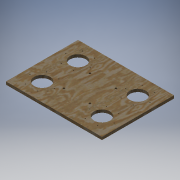
# Autodesk Inventor part: sheetmappingv5
Saved by Autodesk Inventor 2017 (Build 210142000, 142)
## iProperties
Created: 2016-04-30
Part Number: sheetmappingv5
Material: Generic
Document SubType Name: Modeling
Designer: ypatel4
Density: 1 g/cm^3
Appearance: Default
Mass: 4356.33 g
Surface Area: 5620.12 cm^2
Volume: 4356.33 cm^3
Author: ypatel4
Autodesk Inventor part; units mm, degrees
ref_plane "YZ Plane" through (0, 0, 0) normal (1, 0, 0) x (0, 1, 0)
ref_plane "XZ Plane" through (0, 0, 0) normal (0, 1, 0) x (-1, 0, 0)
ref_plane "XY Plane" through (0, 0, 0) normal (0, 0, 1) x (1, 0, 0)
sketch "Sketch1" plane through (0, 0, 0) normal (0, 1, 0) x (-1, 0, 0)
  line L0 (-304.8, 228.6) -> (304.8, 228.6)
  line L1 (304.8, 228.6) -> (304.8, -228.6)
  line L2 (304.8, -228.6) -> (-304.8, -228.6)
  line L3 (-304.8, -228.6) -> (-304.8, 228.6)
  line L4 (-304.8, 228.6) -> (304.8, -228.6) construction
  line L5 (304.8, 228.6) -> (-304.8, -228.6) construction
  line L6 (-304.8, 228.6) -> (304.8, 228.6)
  line L7 (304.8, 228.6) -> (304.8, -228.6)
  line L8 (304.8, -228.6) -> (-304.8, -228.6)
  line L9 (-304.8, -228.6) -> (-304.8, 228.6)
  line L10 (-304.8, 228.6) -> (304.8, -228.6) construction
  line L11 (304.8, 228.6) -> (-304.8, -228.6) construction
  point P0 (0, 0)
  point P1 (0, 0)
  dimension "d0" = 609.6
  dimension "d1" = 457.2
  dimension "d4" = 609.6
  dimension "d5" = 457.2
  constraints: 24 end point, 4 midpoint, 4 parallel, 2 horizontal, 2 perpendicular
  measures "d0" distance of L1.end L2.end
  measures "d1" distance of L0.end L1.end
  measures "d4" distance of L7.end L8.end
  measures "d5" distance of L6.end L7.end
sketch "Sketch2" plane through (0, 0, 0) normal (0, 1, 0) x (-1, 0, 0)
  line L0 (-304.8, 228.6) -> (304.8, 228.6)
  line L1 (304.8, 228.6) -> (304.8, -228.6)
  line L2 (304.8, -228.6) -> (-304.8, -228.6)
  line L3 (-304.8, -228.6) -> (-304.8, 228.6)
  line L4 (-304.8, 228.6) -> (304.8, -228.6) construction
  line L5 (304.8, 228.6) -> (-304.8, -228.6) construction
  circle A0 centre (228.8418, 180.9093) radius 3.175
  circle A1 centre (151.3083, 180.9093) radius 3.175
  circle A2 centre (112.5416, 113.7633) radius 3.175
  circle A3 centre (151.3083, 46.6174) radius 3.175
  circle A4 centre (228.8418, 46.6174) radius 3.175
  circle A5 centre (267.6086, 113.7633) radius 3.175
  circle A6 centre (190.0751, 113.7633) radius 51.1302
  line L6 (-304.8, 228.6) -> (304.8, 228.6)
  line L7 (304.8, 228.6) -> (304.8, -228.6)
  line L8 (304.8, -228.6) -> (-304.8, -228.6)
  line L9 (-304.8, -228.6) -> (-304.8, 228.6)
  line L10 (-304.8, 228.6) -> (304.8, -228.6) construction
  line L11 (304.8, 228.6) -> (-304.8, -228.6) construction
  circle A7 centre (228.8418, 180.9093) radius 3.175
  circle A8 centre (151.3083, 180.9093) radius 3.175
  circle A9 centre (112.5416, 113.7633) radius 3.175
  circle A10 centre (151.3083, 46.6174) radius 3.175
  circle A11 centre (228.8418, 46.6174) radius 3.175
  circle A12 centre (267.6086, 113.7633) radius 3.175
  circle A13 centre (190.0751, 113.7633) radius 51.1302
  point P0 (0, 0)
  point P1 (0, 0)
  point P2 (0, 0)
  dimension "d6" = 609.6
  dimension "d7" = 457.2
  dimension "d8" = 609.6
  dimension "d9" = 457.2
  constraints: 24 end point, 14 centre point, 4 midpoint, 4 parallel, 2 horizontal, 2 perpendicular
  measures "d6" distance of L1.end L2.end
  measures "d7" distance of L0.end L1.end
  measures "d8" distance of L7.end L8.end
  measures "d9" distance of L6.end L7.end
extrude "Extrusion1" add sketch "Sketch1" along normal blind 17.78
sketch "Sketch3" plane through (0, 17.78, 0) normal (0, 1, 0) x (1, 0, 0)
  circle A0 centre (-190.0751, -113.7633) radius 51.1302 projected
  circle A1 centre (-151.3083, -46.6174) radius 3.175 projected
  circle A2 centre (-112.5416, -113.7633) radius 3.175 projected
  circle A3 centre (-151.3083, -180.9093) radius 3.175 projected
  circle A4 centre (-228.8418, -180.9093) radius 3.175 projected
  circle A5 centre (-267.6086, -113.7633) radius 3.175 projected
  circle A6 centre (-228.8418, -46.6174) radius 3.175 projected
  point P0 (0, 0)
hole "Hole1" at (-228.8418, 17.78, 180.9093) at (-267.6086, 17.78, 113.7633) at (-228.8418, 17.78, 46.6174) at (-151.3083, 17.78, 46.6174) at (-112.5416, 17.78, 113.7633) at (-151.3083, 17.78, 180.9093) direction (0, -1, 0) diameter 6.35 end through all
hole "Hole2" at (-190.0751, 0, 113.7633) direction (0, 1, 0) diameter 101.6 depth 46.0375
mirror "Mirror1" about plane through (0, 0, 0) normal (1, 0, 0) of "Hole1", "Hole2"
mirror "Mirror2" about plane through (0, 0, 0) normal (0, 0, 1) of "Hole1", "Hole2", "Mirror1"
sketch "Sketch5" plane through (0, 17.78, 0) normal (0, 1, 0) x (1, 0, 0)
  line L0 (0, 0) -> (82.6543, 82.6543) construction
  line L1 (0, 0) -> (116.8908, 0) construction
  line L2 (0, 0) -> (-82.6543, 82.6543) construction
  line L3 (0, 0) -> (-82.6543, -82.6543) construction
  line L4 (0, 0) -> (116.8908, 0) construction
  line L5 (0, 0) -> (82.6543, -82.6543) construction
  line L6 (0, 0) -> (116.8908, 0) construction
  circle A0 centre (82.6543, 82.6543) radius 6.35
  circle A1 centre (-82.6543, 82.6543) radius 6.35
  circle A2 centre (-82.6543, -82.6543) radius 6.35
  circle A3 centre (82.6543, -82.6543) radius 6.35
  dimension "d41" = 116.8908
  dimension "d42" = 45
  dimension "d43" = 116.8908
  dimension "d44" = 116.8908
  dimension "d45" = 135
  dimension "d46" = 116.8908
  dimension "d47" = 45
  dimension "d48" = 12.7
  dimension "d49" = 12.7
  dimension "d50" = 12.7
  dimension "d51" = 12.7
  constraints: 14 end point, 4 centre point, 4 coincident, 3 equal length, 3 horizontal
  measures "d41" distance of L0.start L0.end
  measures "d42" angle of L1 L0
  measures "d43" distance of L0.start L2.end
  measures "d44" distance of L0.start L3.end
  measures "d45" angle of L3 L4
  measures "d46" distance of L0.start L5.end
  measures "d47" angle of L5 L6
  measures "d48" diameter of A0
  measures "d49" diameter of A1
  measures "d50" diameter of A2
  measures "d51" diameter of A3
hole "Hole4" at (82.6543, 17.78, -82.6543) at (82.6543, 17.78, 82.6543) at (-82.6543, 17.78, 82.6543) at (-82.6543, 17.78, -82.6543) direction (0, -1, 0) diameter 12.7 end through all
body "Solid1"
